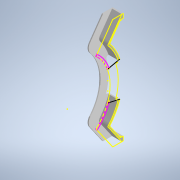
# Autodesk Inventor part: vydacha_backstenka
Saved by Autodesk Inventor 2022 (Build 260153000, 153)
## iProperties
Created: 2024-09-10
Part Number: vydacha_backstenka
Material: Типовые
Document SubType Name: Modeling
Designer: Andrey
Density: 1 g/cm^3
Appearance: По умолчанию
Author: Andrey
Autodesk Inventor part; units mm, degrees
ref_plane "YZ Plane" through (0, 0, 0) normal (1, 0, 0) x (0, 1, 0)
ref_plane "XZ Plane" through (0, 0, 0) normal (0, 1, 0) x (-1, 0, 0)
sketch "Эскиз6" plane through (0, 0, 0) normal (1, 0, 0) x (0, 1, 0)
  circle A0 centre (0, 0) radius 59
  arc A1 (-43.5, -52.2661) -> (43.5, -52.2661) centre (0, 0) ccw
  arc A2 (-33.2647, -39.9682) -> (-18.3457, -48.6563) centre (0, 0) ccw
  line L0 (-5.5, -64.5) -> (5.5, -64.5)
  line L1 (5.5, -53.5) -> (-5.5, -53.5)
  circle A3 centre (0, 0) radius 53.5
  circle A4 centre (0, 0) radius 64.7341
  line L2 (66.7947, -70.548) -> (66.7947, -67.5)
  line L3 (-66.7947, -70.548) -> (-66.7947, -67.5)
  line L4 (-64.1174, -67.5) -> (-66.7947, -67.5)
  line L5 (66.7947, -67.5) -> (64.1174, -67.5)
  line L6 (-66.7947, -67.5) -> (-41.4303, -49.7396)
  line L7 (66.7947, -67.5) -> (41.4303, -49.7396)
  line L8 (-64.1796, -67.5) -> (-40.22, -50.7233)
  line L9 (64.1796, -67.5) -> (40.22, -50.7233)
  line L10 (-60.7947, -119.148) -> (-60.7947, -81.948)
  line L11 (-60.7947, -100.548) -> (-60.7947, -65.548)
  line L12 (-60.7947, -65.548) -> (-48.7947, -65.548)
  line L13 (-48.7947, -65.548) -> (-48.7947, -100.548)
  line L14 (-48.7947, -100.548) -> (-60.7947, -100.548)
  line L15 (-47.7947, -64.548) -> (-61.7947, -64.548)
  line L16 (-61.7947, -64.548) -> (-61.7947, -101.548)
  line L17 (-61.7947, -101.548) -> (-47.7947, -101.548)
  line L18 (-47.7947, -101.548) -> (-47.7947, -64.548)
  line L19 (-66.7947, -65.6688) -> (-42.6089, -48.7338)
  line L20 (-66.7947, -65.6688) -> (-66.7947, -67.5)
  line L21 (66.7947, -65.6688) -> (42.6089, -48.7338)
  line L22 (66.7947, -65.6688) -> (66.7947, -67.5)
  arc A5 (10.4469, -65.8979) -> (12.7447, -66.3164) centre (12.091, -63.3885) ccw
  line L23 (12.7447, -66.3164) -> (16.61, -65.4535)
  arc A6 (16.61, -65.4535) -> (18.5547, -64.025) centre (15.9563, -62.5255) ccw
  arc A7 (19.9415, -62.6063) -> (18.5547, -64.025) centre (22.0192, -66.0244) ccw
  arc A8 (19.9415, -62.6063) -> (20.398, -61.5339) centre (19.4221, -61.7518) ccw
  line L24 (20.398, -61.5339) -> (17.9394, -50.5215)
  arc A9 (17.9394, -50.5215) -> (17.0312, -49.7417) centre (16.9635, -50.7394) ccw
  arc A10 (15.2478, -49.1829) -> (17.0312, -49.7417) centre (17.3024, -45.7509) ccw
  arc A11 (15.2478, -49.1829) -> (13.0531, -48.829) centre (13.7068, -51.757) ccw
  line L25 (13.0531, -48.829) -> (8.6292, -49.8167)
  arc A12 (8.6292, -49.8167) -> (7.1584, -50.6265) centre (9.2829, -52.7446) ccw
  arc A13 (4.0448, -50.9698) -> (7.1584, -50.6265) centre (5.388, -48.8613) ccw
  arc A14 (4.0448, -50.9698) -> (2.4329, -50.5) centre (2.4329, -53.5) ccw
  line L26 (2.4329, -50.5) -> (-2.4329, -50.5)
  arc A15 (-2.4329, -50.5) -> (-4.0448, -50.9698) centre (-2.4329, -53.5) ccw
  arc A16 (-7.1584, -50.6265) -> (-4.0448, -50.9698) centre (-5.388, -48.8613) ccw
  arc A17 (-7.1584, -50.6265) -> (-8.6292, -49.8167) centre (-9.2829, -52.7446) ccw
  line L27 (-8.6292, -49.8167) -> (-13.0531, -48.829)
  arc A18 (-13.0531, -48.829) -> (-15.2478, -49.1829) centre (-13.7068, -51.757) ccw
  arc A19 (-17.0312, -49.7417) -> (-15.2478, -49.1829) centre (-17.3024, -45.7509) ccw
  arc A20 (-17.0312, -49.7417) -> (-17.9394, -50.5215) centre (-16.9635, -50.7394) ccw
  line L28 (-17.9394, -50.5215) -> (-20.398, -61.5339)
  arc A21 (-20.398, -61.5339) -> (-19.9415, -62.6063) centre (-19.4221, -61.7518) ccw
  arc A22 (-18.5547, -64.025) -> (-19.9415, -62.6063) centre (-22.0192, -66.0244) ccw
  arc A23 (-18.5547, -64.025) -> (-16.61, -65.4535) centre (-15.9563, -62.5255) ccw
  line L29 (-16.61, -65.4535) -> (-12.7447, -66.3164)
  arc A24 (-12.7447, -66.3164) -> (-10.4469, -65.8979) centre (-12.091, -63.3885) ccw
  arc A25 (-7.7813, -65.2719) -> (-10.4469, -65.8979) centre (-8.2548, -69.2438) ccw
  arc A26 (-7.7813, -65.2719) -> (-6.628, -65.3991) centre (0, 0) ccw
  arc A27 (-4.1629, -66.5909) -> (-6.628, -65.3991) centre (-7.0314, -69.3787) ccw
  arc A28 (-4.1629, -66.5909) -> (-2.0116, -67.5) centre (-2.0116, -64.5) ccw
  line L30 (-2.0116, -67.5) -> (2.0116, -67.5)
  arc A29 (2.0116, -67.5) -> (4.1629, -66.5909) centre (2.0116, -64.5) ccw
  arc A30 (6.628, -65.3991) -> (4.1629, -66.5909) centre (7.0314, -69.3787) ccw
  arc A31 (6.628, -65.3991) -> (7.7813, -65.2719) centre (0, 0) ccw
  arc A32 (10.4469, -65.8979) -> (7.7813, -65.2719) centre (8.2548, -69.2438) ccw
  line L31 (-12.0455, -60.8371) -> (-14.9734, -60.1834)
  arc A33 (-16.1106, -58.3926) -> (-14.9734, -60.1834) centre (-14.6466, -58.7195) ccw
  line L32 (-16.1106, -58.3926) -> (-15.4569, -55.4647)
  arc A34 (-13.6661, -54.3276) -> (-15.4569, -55.4647) centre (-13.9929, -55.7916) ccw
  line L33 (-13.6661, -54.3276) -> (-10.7382, -54.9813)
  arc A35 (-9.601, -56.7721) -> (-10.7382, -54.9813) centre (-11.065, -56.4452) ccw
  line L34 (-9.601, -56.7721) -> (-10.2547, -59.7)
  arc A36 (-12.0455, -60.8371) -> (-10.2547, -59.7) centre (-11.7187, -59.3732) ccw
  line L35 (3, -57.5) -> (3, -60.5)
  arc A37 (1.5, -62) -> (3, -60.5) centre (1.5, -60.5) ccw
  line L36 (1.5, -62) -> (-1.5, -62)
  arc A38 (-3, -60.5) -> (-1.5, -62) centre (-1.5, -60.5) ccw
  line L37 (-3, -60.5) -> (-3, -57.5)
  arc A39 (-1.5, -56) -> (-3, -57.5) centre (-1.5, -57.5) ccw
  line L38 (-1.5, -56) -> (1.5, -56)
  arc A40 (3, -57.5) -> (1.5, -56) centre (1.5, -57.5) ccw
  line L39 (14.9734, -60.1834) -> (12.0455, -60.8371)
  arc A41 (10.2547, -59.7) -> (12.0455, -60.8371) centre (11.7187, -59.3732) ccw
  line L40 (10.2547, -59.7) -> (9.601, -56.7721)
  arc A42 (10.7382, -54.9813) -> (9.601, -56.7721) centre (11.065, -56.4452) ccw
  line L41 (10.7382, -54.9813) -> (13.6661, -54.3276)
  arc A43 (15.4569, -55.4647) -> (13.6661, -54.3276) centre (13.9929, -55.7916) ccw
  line L42 (15.4569, -55.4647) -> (16.1106, -58.3926)
  arc A44 (14.9734, -60.1834) -> (16.1106, -58.3926) centre (14.6466, -58.7195) ccw
  line L43 (-17.5874, -48.9448) -> (-17.9148, -50.4114)
  line L44 (-17.4757, -48.4443) -> (-17.5874, -48.9448)
  arc A45 (-17.4757, -48.4443) -> (-16.5671, -48.7625) centre (0, 0) ccw
  line L45 (17.5874, -48.9448) -> (17.9148, -50.4114)
  line L46 (17.5874, -48.9448) -> (17.4757, -48.4443)
  arc A46 (16.5671, -48.7625) -> (17.4757, -48.4443) centre (0, 0) ccw
  spline S0 degree 3 poles (16.5671, -48.7625) (16.4879, -48.7894) (16.4083, -48.8162) (16.0592, -48.933) (15.871, -48.9937) (15.6206, -49.0741) (15.5161, -49.1071) (15.3732, -49.152) (15.3217, -49.168) (15.2685, -49.1846) (15.2566, -49.1883) (15.2567, -49.1883) knots 0 0 0 0 0.082005 0.082005 0.358696 0.358696 0.636163 0.636163 0.853047 0.853047 1 1 1 1
  arc A47 (-13.8029, -50.3511) -> (-14.3262, -49.4673) centre (-14.5349, -50.1876) ccw
  line L47 (-13.8029, -50.3511) -> (-13.8664, -50.6357)
  arc A48 (-17.6953, -49.428) -> (-13.8664, -50.6357) centre (0, 0) ccw
  line L48 (-17.6953, -49.428) -> (-17.4757, -48.4443)
  arc A49 (-17.4757, -48.4443) -> (-14.3262, -49.4673) centre (0, 0) ccw
  arc A50 (14.3262, -49.4673) -> (13.8029, -50.3511) centre (14.5349, -50.1876) ccw
  arc A51 (14.3262, -49.4673) -> (17.4757, -48.4443) centre (0, 0) ccw
  line L49 (17.4757, -48.4443) -> (17.6953, -49.428)
  arc A52 (13.8664, -50.6357) -> (17.6953, -49.428) centre (0, 0) ccw
  line L50 (13.8664, -50.6357) -> (13.8029, -50.3511)
  arc A53 (20.0103, -63.6634) -> (20.8157, -63.4046) centre (0, 0) ccw
  line L51 (20.7501, -63.1106) -> (20.398, -61.5339)
  line L52 (20.8157, -63.4046) -> (20.7501, -63.1106)
  line L53 (-20.398, -61.5339) -> (-20.7501, -63.1106)
  line L54 (-20.7501, -63.1106) -> (-20.8157, -63.4046)
  arc A54 (-20.8157, -63.4046) -> (-20.0103, -63.6634) centre (0, 0) ccw
  spline S1 degree 3 poles (-20.0103, -63.6634) (-19.7276, -63.7522) (-19.4173, -63.8474) (-18.9718, -63.9808) (-18.8458, -64.0178) (-18.7115, -64.0571) (-18.6753, -64.0677) (-18.6443, -64.0767) knots 0 0 0 0 0.535332 0.535332 0.857412 0.857412 1 1 1 1
  circle A55 centre (0, 0) radius 66.7341
  circle A56 centre (0, 0) radius 51.5
  line L55 (-17.4757, -48.4443) -> (-20.8157, -63.4046)
  line L56 (17.4757, -48.4443) -> (20.8157, -63.4046)
  line L57 (17.7126, -48.3582) -> (21.0542, -63.3258)
  line L58 (-17.7126, -48.3582) -> (-21.0542, -63.3258)
  line L59 (66.7947, -65.6688) -> (66.7947, -54.6688)
  line L60 (66.7947, -54.6688) -> (38.1409, -34.6052)
  line L61 (-66.7947, -65.6688) -> (-66.7947, -54.6688)
  line L62 (-66.7947, -54.6688) -> (-38.1409, -34.6052)
  arc A57 (-20.334, -61.2469) -> (-16.491, -62.3914) centre (0, 0) ccw
  line L63 (-16.5346, -62.5868) -> (-16.491, -62.3914)
  arc A58 (-16.5346, -62.5868) -> (-16.4618, -62.606) centre (0, 0) ccw
  arc A59 (-14.251, -61.6073) -> (-16.4618, -62.606) centre (-14.7017, -63.5558) ccw
  arc A60 (-14.251, -61.6073) -> (-13.3049, -61.8185) centre (0, 0) ccw
  arc A61 (-11.7289, -63.6627) -> (-13.3049, -61.8185) centre (-13.7258, -63.7737) ccw
  arc A62 (-11.7289, -63.6627) -> (-11.6548, -63.6763) centre (0, 0) ccw
  line L64 (-11.6112, -63.4809) -> (-11.6548, -63.6763)
  arc A63 (-11.6112, -63.4809) -> (-2.5, -64.4856) centre (0, 0) ccw
  line L65 (-2.5, -64.6858) -> (-2.5, -64.4856)
  arc A64 (-2.5, -64.6858) -> (-2.4247, -64.6886) centre (0, 0) ccw
  arc A65 (-0.4847, -63.2322) -> (-2.4247, -64.6886) centre (-0.5, -65.2322) ccw
  arc A66 (-0.4847, -63.2322) -> (0.4847, -63.2322) centre (0, 0) ccw
  arc A67 (2.4247, -64.6886) -> (0.4847, -63.2322) centre (0.5, -65.2322) ccw
  arc A68 (2.4247, -64.6886) -> (2.5, -64.6858) centre (0, 0) ccw
  line L66 (2.5, -64.4856) -> (2.5, -64.6858)
  arc A69 (2.5, -64.4856) -> (11.6112, -63.4809) centre (0, 0) ccw
  line L67 (11.6548, -63.6763) -> (11.6112, -63.4809)
  arc A70 (11.6548, -63.6763) -> (11.7289, -63.6627) centre (0, 0) ccw
  arc A71 (13.3049, -61.8185) -> (11.7289, -63.6627) centre (13.7258, -63.7737) ccw
  arc A72 (13.3049, -61.8185) -> (14.251, -61.6073) centre (0, 0) ccw
  arc A73 (16.4618, -62.606) -> (14.251, -61.6073) centre (14.7017, -63.5558) ccw
  arc A74 (16.4618, -62.606) -> (16.5346, -62.5868) centre (0, 0) ccw
  line L68 (16.491, -62.3914) -> (16.5346, -62.5868)
  arc A75 (16.491, -62.3914) -> (20.334, -61.2469) centre (0, 0) ccw
  line L69 (20.1965, -60.6311) -> (20.334, -61.2469)
  arc A76 (-17.672, -59.1506) -> (17.672, -59.1506) centre (0, 0) ccw
  line L70 (-20.334, -61.2469) -> (-20.1965, -60.6311)
  circle A77 centre (0, 0) radius 61.7341
  circle A78 centre (0, 0) radius 61.3341
  arc A79 (-17.672, -59.1506) -> (-20.1965, -60.6311) centre (-18.2445, -61.0669) ccw
  arc A80 (20.1965, -60.6311) -> (17.672, -59.1506) centre (18.2445, -61.0669) ccw
  line L71 (-66.7947, -67.5) -> (-61.7947, -67.5)
  line L72 (-61.7947, -67.5) -> (-61.7947, -63.999)
  line L73 (66.7947, -67.5) -> (61.7947, -67.5)
  line L74 (61.7947, -67.5) -> (61.7947, -62.1678)
  point P0 (-43.1262, -50.9271)
  point P1 (43.1262, -50.9271)
  point P2 (19.7206, -58.4995)
  point P3 (-19.7206, -58.4995)
  point P4 (-17.9089, -50.4135)
  point P5 (-17.9394, -50.5215)
  point P6 (-17.9148, -50.4114)
  point P7 (14.3262, -49.4673)
  point P8 (6.5324, -51.084)
  point P9 (4.7555, -51.28)
  point P10 (-4.7555, -51.28)
  point P11 (-6.5324, -51.084)
  point P12 (-14.3262, -49.4673)
  point P13 (-19.871, -58.026)
  point P14 (19.871, -58.026)
  point P15 (17.9089, -50.4135)
  point P16 (17.9148, -50.4114)
  point P17 (61.7947, -63.999)
  dimension "d18" = 118
  dimension "d19" = 35
  dimension "d20" = 35
  dimension "d21" = 1.5
  dimension "d22" = 1.5
  dimension "d23" = 35
  dimension "d24" = 12
  dimension "d25" = 1
  dimension "d26" = 1.5
  dimension "d27" = 1.5
  dimension "d28" = 0.25
  dimension "d29" = 0.25
  dimension "d30" = 11
  dimension "d31" = 11
  dimension "d34" = 0.4
  dimension "d36" = 5
  dimension "d37" = 5
  constraints: 56 end point, 10 point on line, 8 parallel, 8 point on circle, 5 centre point, 5 coincident, 5 perpendicular, 4 vertical, 1 collinear, 1 horizontal, 1 midpoint, 1 tangent, 15 other
  measures "d18" diameter of A0
  measures "d19" angle of L7 L5
  measures "d20" angle of L4 L6
  measures "d21" distance between parallel lines of L6 L8
  measures "d22" distance between parallel lines of L7 L9
  measures "d23" distance of L11.start L11.end
  measures "d24" distance of L11.end L12.end
  measures "d25" distance between parallel lines of L12 L15
  measures "d26" distance between parallel lines of L6 L19
  measures "d27" distance between parallel lines of L7 L21
  measures "d28" distance between parallel lines of L56 L57
  measures "d29" distance between parallel lines of L55 L58
  measures "d30" distance of L21.start L59.end
  measures "d31" distance of L19.start L61.end
  measures "d36" distance of L3.end L71.end
  measures "d37" distance of L2.end L73.end
extrude "Выдавливание5" add sketch "Эскиз6" along normal blind 1.2 contours L62 A3 L58 A0 | A0 L58 A78 L62 | L60 A78 L57 A0 | A0 L57 A3 L60 | L58 A3 L55 L28 A0 | A0 L28 A78 L58 | A78 L58 A77 L62 | L62 A56 L58 A3 | L57 A78 L24 A0 | A0 L24 L56 A3 L57 | L60 A77 L57 A78 | A3 L57 A56 L60 | L28 A20 A3 A9 L24 A0 L42 A43 L41 A42 L40 L35 A40 L38 A39 L37 L34 A35 L33 A34 L32 | A0 L32 A33 A78 L28 | L58 A56 L44 L43 A3 | A77 L58 A4 L62 | L24 A78 A44 L42 A0 | A3 L45 L46 A56 L57 | L60 A4 L57 A77 | L32 A34 L33 A35 L34 A0 | A0 L34 A36 A78 A33 L32 | L43 A48 A19 A20 A3 | A4 L19 A55 L62 | L42 A44 A78 A41 L40 A0 | A0 L40 A42 L41 A43 L42 | A3 A9 A10 A52 L45 | L60 A55 L21 A4 | A0 L37 A38 A78 A36 L34 | A20 A19 A48 L47 A47 A56 A16 A13 A50 L50 A52 A10 A9 A3 | L43 L44 A45 A49 A19 A48 | L58 A55 L8 A4 | A4 L6 A55 L19 | A55 L19 L61 L62 | L40 A41 A78 A37 L35 A0 | A52 A10 S0 A46 L46 L45 | A4 L9 A55 L57 | L21 A55 L7 A4 | L60 L59 L21 A55 | L37 A39 L38 A40 L35 A0 | A0 L35 A37 A78 A38 L37 | A19 A49 A47 L47 A48 | L8 A55 L6 A4 | A55 L6 L20 L19 | A52 L50 A50 A51 A10 | A4 L7 A55 L9 | L21 L74 L7 A55 | L21 L22 L7 L74 | L72 L16 L8 L4 L6 | L7 L5 L9 L74 | L8 L16 L71 L4 | L9 L5 L73 L74
fillet "Сопряжение1" radius 2 2 edges at (0.6, 19.871, -58.026) (0.6, -19.871, -58.026)
fillet "Сопряжение2" radius 1 2 edges at (0.6, 61.7947, -63.999) (0.6, -61.7947, -63.999)
sketch "Эскиз7" plane through (1.2, 0, 0) normal (1, 0, 0) x (0, 0, -1)
  arc A0 (34.6052, -38.1409) -> (51.084, -6.5324) centre (0, 0) ccw projected
  line L0 (34.6052, -38.1409) -> (54.6688, -66.7947) projected
  line L1 (54.6688, -66.7947) -> (67.5, -66.7947) projected
  line L2 (67.5, -66.7947) -> (67.5, -61.7947) projected
  line L3 (67.5, -61.7947) -> (64.5195, -61.7947) projected
  arc A1 (63.7004, -61.3683) -> (64.5195, -61.7947) centre (64.5195, -60.7947) ccw projected
  line L4 (63.7004, -61.3683) -> (50.9271, -43.1262) projected
  arc A2 (50.9271, -43.1262) -> (63.3258, -21.0542) centre (0, 0) ccw projected
  line L5 (63.3258, -21.0542) -> (60.1674, -20.3491) projected
  arc A3 (58.6894, -17.8162) -> (60.1674, -20.3491) centre (60.6032, -18.3972) ccw projected
  arc A4 (58.6894, -17.8162) -> (58.6894, 17.8162) centre (0, 0) ccw projected
  arc A5 (60.1674, 20.3491) -> (58.6894, 17.8162) centre (60.6032, 18.3972) ccw projected
  line L6 (60.1674, 20.3491) -> (63.3258, 21.0542) projected
  arc A6 (63.3258, 21.0542) -> (50.9271, 43.1262) centre (0, 0) ccw projected
  line L7 (50.9271, 43.1262) -> (63.7004, 61.3683) projected
  arc A7 (64.5195, 61.7947) -> (63.7004, 61.3683) centre (64.5195, 60.7947) ccw projected
  line L8 (64.5195, 61.7947) -> (67.5, 61.7947) projected
  line L9 (67.5, 61.7947) -> (67.5, 66.7947) projected
  line L10 (67.5, 66.7947) -> (54.6688, 66.7947) projected
  line L11 (54.6688, 66.7947) -> (34.6052, 38.1409) projected
  arc A8 (51.084, 6.5324) -> (34.6052, 38.1409) centre (0, 0) ccw projected
  arc A9 (51.28, 4.7555) -> (51.084, 6.5324) centre (48.8613, 5.388) ccw projected
  arc A10 (51.28, -4.7555) -> (51.28, 4.7555) centre (0, 0) ccw projected
  arc A11 (51.084, -6.5324) -> (51.28, -4.7555) centre (48.8613, -5.388) ccw projected
  arc A12 (50.4135, -17.9089) -> (50.5215, -17.9394) centre (50.7394, -16.9635) ccw projected
  line L12 (50.5215, -17.9394) -> (50.4114, -17.9148) projected
  arc A13 (50.4114, -17.9148) -> (50.4135, -17.9089) centre (0, 0) ccw projected
  arc A14 (50.4135, 17.9089) -> (50.4114, 17.9148) centre (0, 0) ccw projected
  line L13 (50.4114, 17.9148) -> (50.5215, 17.9394) projected
  arc A15 (50.5215, 17.9394) -> (50.4135, 17.9089) centre (50.7394, 16.9635) ccw projected
  line L14 (54.6688, -66.7947) -> (67.5, -66.7947) projected
  line L15 (65.6688, -66.7947) -> (49.9141, -44.2947)
  arc A16 (34.6052, -38.1409) -> (51.084, -6.5324) centre (0, 0) ccw projected
  line L16 (63.7004, -61.3683) -> (50.9271, -43.1262) projected
  circle A17 centre (0, 0) radius 66.7341
  line L17 (49.9141, 44.2947) -> (65.6688, 66.7947)
  line L18 (67.5, 66.7947) -> (54.6688, 66.7947) projected
  arc A18 (62.4711, 16.9666) -> (61.443, 20.3778) centre (0, 0) ccw projected
  circle A19 centre (0, 0) radius 64.7341
  line L19 (49.9141, 44.2947) -> (48.7338, 42.6089)
  line L20 (49.9141, -44.2947) -> (48.7338, -42.6089)
  line L21 (63.3258, -21.0542) -> (60.1674, -20.3491) projected
  line L22 (63.3258, -21.0542) -> (48.3582, -17.7126)
  line L23 (63.3258, 21.0542) -> (48.3582, 17.7126)
  arc A20 (51.084, 6.5324) -> (34.6052, 38.1409) centre (0, 0) ccw projected
  arc A21 (50.4135, -17.9089) -> (51.4548, -14.651) centre (0, 0) ccw
  circle A22 centre (0, 0) radius 53.5
  point P0 (0, 0)
  point P1 (61.3635, -20.6161)
  point P2 (61.3635, 20.6161)
  point P3 (35.7612, -39.7918)
  point P4 (50.3265, -18.152)
  point P5 (50.3265, 18.152)
  point P6 (35.7612, 39.7918)
  dimension "d39" = 1.5
  dimension "d40" = 1.5
  constraints: 12 end point, 10 point on circle, 4 collinear, 3 centre point, 3 coincident, 2 parallel, 2 point on line, 7 other
  measures "d39" distance between parallel lines of L16 L15
  measures "d40" distance between parallel lines of L7 L17
ref_plane "РабПлоскость1" through (11.9, 16.1346, -61.6905) normal (-1, 0, 0) x (0, 0, 1)
extrude "Выдавливание6" add sketch "Эскиз7" along normal blind 11.5 contours A19 L5 A2 A17 L20 | A17 L4 A1 L3 L2 L1 L15 | L19 A17 A6 L6 A19 | L17 L10 L9 L8 A7 L7 A17
sketch "Эскиз9" plane through (12.7, 0, 0) normal (1, 0, 0) x (0, 0, -1)
  arc A0 (50.4135, 17.9089) -> (50.4114, 17.9148) centre (0, 0) ccw projected
  line L0 (50.4114, 17.9148) -> (50.5215, 17.9394) projected
  arc A1 (50.5215, 17.9394) -> (50.4135, 17.9089) centre (50.7394, 16.9635) ccw projected
  arc A2 (50.4135, -17.9089) -> (50.5215, -17.9394) centre (50.7394, -16.9635) ccw projected
  line L1 (50.5215, -17.9394) -> (50.4114, -17.9148) projected
  arc A3 (50.4114, -17.9148) -> (50.4135, -17.9089) centre (0, 0) ccw projected
  arc A4 (61.3635, 20.6161) -> (48.7338, 42.6089) centre (0, 0) ccw projected
  line L2 (48.7338, 42.6089) -> (65.6688, 66.7947) projected
  line L3 (65.6688, 66.7947) -> (54.6688, 66.7947) projected
  line L4 (54.6688, 66.7947) -> (34.6052, 38.1409) projected
  arc A5 (51.084, 6.5324) -> (34.6052, 38.1409) centre (0, 0) ccw projected
  arc A6 (51.28, 4.7555) -> (51.084, 6.5324) centre (48.8613, 5.388) ccw projected
  arc A7 (51.28, -4.7555) -> (51.28, 4.7555) centre (0, 0) ccw projected
  arc A8 (51.084, -6.5324) -> (51.28, -4.7555) centre (48.8613, -5.388) ccw projected
  arc A9 (34.6052, -38.1409) -> (51.084, -6.5324) centre (0, 0) ccw projected
  line L5 (34.6052, -38.1409) -> (54.6688, -66.7947) projected
  line L6 (54.6688, -66.7947) -> (65.6688, -66.7947) projected
  line L7 (65.6688, -66.7947) -> (48.7338, -42.6089) projected
  arc A10 (48.7338, -42.6089) -> (61.3635, -20.6161) centre (0, 0) ccw projected
  line L8 (61.3635, -20.6161) -> (60.1674, -20.3491) projected
  arc A11 (58.6894, -17.8162) -> (60.1674, -20.3491) centre (60.6032, -18.3972) ccw projected
  arc A12 (58.6894, -17.8162) -> (58.6894, 17.8162) centre (0, 0) ccw projected
  arc A13 (60.1674, 20.3491) -> (58.6894, 17.8162) centre (60.6032, 18.3972) ccw projected
  line L9 (60.1674, 20.3491) -> (61.3635, 20.6161) projected
  line L10 (35.7612, 39.7918) -> (34.6052, 38.1409) projected
  arc A14 (48.3582, 17.7126) -> (34.6052, 38.1409) centre (0, 0) ccw projected
  line L11 (48.3582, 17.7126) -> (50.3265, 18.152) projected
  arc A15 (50.3265, 18.152) -> (35.7612, 39.7918) centre (0, 0) ccw projected
  line L12 (50.3265, -18.152) -> (48.3582, -17.7126) projected
  arc A16 (34.6052, -38.1409) -> (48.3582, -17.7126) centre (0, 0) ccw projected
  line L13 (34.6052, -38.1409) -> (35.7612, -39.7918) projected
  arc A17 (35.7612, -39.7918) -> (50.3265, -18.152) centre (0, 0) ccw projected
  line L14 (67.5, -61.7947) -> (64.5195, -61.7947) projected
  arc A18 (63.7004, -61.3683) -> (64.5195, -61.7947) centre (64.5195, -60.7947) ccw projected
  line L15 (63.7004, -61.3683) -> (50.9271, -43.1262) projected
  arc A19 (50.9271, -43.1262) -> (63.3258, -21.0542) centre (0, 0) ccw projected
  line L16 (63.3258, -21.0542) -> (61.3635, -20.6161) projected
  arc A20 (48.7338, -42.6089) -> (61.3635, -20.6161) centre (0, 0) ccw projected
  line L17 (48.7338, -42.6089) -> (65.6688, -66.7947) projected
  line L18 (65.6688, -66.7947) -> (67.5, -66.7947) projected
  line L19 (67.5, -66.7947) -> (67.5, -61.7947) projected
  arc A21 (61.3635, 20.6161) -> (48.7338, 42.6089) centre (0, 0) ccw projected
  line L20 (61.3635, 20.6161) -> (63.3258, 21.0542) projected
  arc A22 (63.3258, 21.0542) -> (50.9271, 43.1262) centre (0, 0) ccw projected
  line L21 (50.9271, 43.1262) -> (63.7004, 61.3683) projected
  arc A23 (64.5195, 61.7947) -> (63.7004, 61.3683) centre (64.5195, 60.7947) ccw projected
  line L22 (64.5195, 61.7947) -> (67.5, 61.7947) projected
  line L23 (67.5, 61.7947) -> (67.5, 66.7947) projected
  line L24 (67.5, 66.7947) -> (65.6688, 66.7947) projected
  line L25 (65.6688, 66.7947) -> (48.7338, 42.6089) projected
  line L26 (63.3258, -21.0542) -> (60.1674, -20.3491) projected
  line L27 (63.3258, -21.0542) -> (48.3582, -17.7126)
  line L28 (48.3582, 17.7126) -> (63.3258, 21.0542)
  point P0 (0, 0)
  constraints: 4 end point, 1 collinear
fillet "Сопряжение3" radius 5 4 edges at (6.95, -42.6089, -48.7338) (6.35, -43.1262, -50.9271) (6.35, 43.1262, -50.9271) (6.95, 42.6089, -48.7338)
sketch "Эскиз10" plane through (0, 0, 0) normal (-1, 0, 0) x (0, 0, 1)
  arc A0 (-51.084, -6.5324) -> (-34.6052, -38.1409) centre (0, 0) ccw projected
  arc A1 (-51.28, -4.7555) -> (-51.084, -6.5324) centre (-48.8613, -5.388) ccw projected
  arc A2 (-51.28, 4.7555) -> (-51.28, -4.7555) centre (0, 0) ccw projected
  arc A3 (-51.084, 6.5324) -> (-51.28, 4.7555) centre (-48.8613, 5.388) ccw projected
  arc A4 (-34.6052, 38.1409) -> (-51.084, 6.5324) centre (0, 0) ccw projected
  line L0 (-54.6688, 66.7947) -> (-34.6052, 38.1409) projected
  line L1 (-67.5, 66.7947) -> (-54.6688, 66.7947) projected
  line L2 (-67.5, 61.7947) -> (-67.5, 66.7947) projected
  line L3 (-64.5195, 61.7947) -> (-67.5, 61.7947) projected
  arc A5 (-63.7004, 61.3683) -> (-64.5195, 61.7947) centre (-64.5195, 60.7947) ccw projected
  line L4 (-53.0756, 46.1946) -> (-63.7004, 61.3683) projected
  arc A6 (-53.1865, 40.3068) -> (-53.0756, 46.1946) centre (-57.1714, 43.3267) ccw projected
  arc A7 (-53.1865, 40.3068) -> (-63.3258, 21.0542) centre (0, 0) ccw projected
  line L5 (-60.1674, 20.3491) -> (-63.3258, 21.0542) projected
  arc A8 (-58.6894, 17.8162) -> (-60.1674, 20.3491) centre (-60.6032, 18.3972) ccw projected
  arc A9 (-58.6894, 17.8162) -> (-58.6894, -17.8162) centre (0, 0) ccw projected
  arc A10 (-60.1674, -20.3491) -> (-58.6894, -17.8162) centre (-60.6032, -18.3972) ccw projected
  line L6 (-63.3258, -21.0542) -> (-60.1674, -20.3491) projected
  arc A11 (-63.3258, -21.0542) -> (-53.1865, -40.3068) centre (0, 0) ccw projected
  arc A12 (-53.0756, -46.1946) -> (-53.1865, -40.3068) centre (-57.1714, -43.3267) ccw projected
  line L7 (-63.7004, -61.3683) -> (-53.0756, -46.1946) projected
  arc A13 (-64.5195, -61.7947) -> (-63.7004, -61.3683) centre (-64.5195, -60.7947) ccw projected
  line L8 (-67.5, -61.7947) -> (-64.5195, -61.7947) projected
  line L9 (-67.5, -66.7947) -> (-67.5, -61.7947) projected
  line L10 (-54.6688, -66.7947) -> (-67.5, -66.7947) projected
  line L11 (-34.6052, -38.1409) -> (-54.6688, -66.7947) projected
  arc A14 (-50.5215, -17.9394) -> (-50.4135, -17.9089) centre (-50.7394, -16.9635) ccw projected
  arc A15 (-50.4135, -17.9089) -> (-50.4114, -17.9148) centre (0, 0) ccw projected
  line L12 (-50.5215, -17.9394) -> (-50.4114, -17.9148) projected
  arc A16 (-50.4114, 17.9148) -> (-50.4135, 17.9089) centre (0, 0) ccw projected
  arc A17 (-50.4135, 17.9089) -> (-50.5215, 17.9394) centre (-50.7394, 16.9635) ccw projected
  line L13 (-50.4114, 17.9148) -> (-50.5215, 17.9394) projected
  arc A18 (-51.0665, 39.7834) -> (-50.915, 45.7241) centre (-55.0108, 42.8562) ccw projected
  line L14 (-48.7338, 42.6089) -> (-65.6688, 66.7947) projected
  line L15 (-48.7338, 42.6089) -> (-40.8542, 31.3558)
  arc A19 (-34.6052, 38.1409) -> (-51.084, 6.5324) centre (0, 0) ccw projected
  line L16 (-65.6688, -66.7947) -> (-48.7338, -42.6089) projected
  line L17 (-48.7338, -42.6089) -> (-40.8542, -31.3558)
  circle A20 centre (-46.2336, 39.0384) radius 9.0107
  circle A21 centre (-46.2336, -39.0384) radius 9.0107
  line L18 (-54.6688, 66.7947) -> (-34.6052, 38.1409) projected
  point P0 (0, 0)
  point P1 (-38.8525, -44.2067)
  point P2 (-39.3489, -33.2251)
  point P3 (-39.3489, 33.2251)
  point P4 (-38.8525, 44.2067)
  constraints: 4 end point, 4 tangent, 2 centre point, 2 collinear, 2 point on circle, 2 point on line
extrude "Выдавливание8" cut sketch "Эскиз10" against normal blind 15 contours A0 L11 A21 | A20 L0 A4
